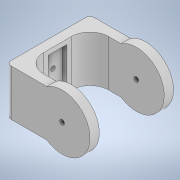
# Autodesk Inventor part: PartArm1
Saved by Autodesk Inventor 2022 (Build 260153000, 153)
## iProperties
Created: 2022-01-07
Part Number: PartArm1
Material: Generic
Document SubType Name: Modeling
Designer: nguye
Density: 1 g/cm^3
Appearance: Default
Author: nguye
Autodesk Inventor part; units mm, degrees
ref_plane "YZ Plane" through (0, 0, 0) normal (1, 0, 0) x (0, 1, 0)
ref_plane "XZ Plane" through (0, 0, 0) normal (0, 1, 0) x (-1, 0, 0)
ref_plane "XY Plane" through (0, 0, 0) normal (0, 0, 1) x (1, 0, 0)
sketch "Sketch1" plane through (0, 0, 0) normal (0, 1, 0) x (-1, 0, 0)
  line L0 (45, 0) -> (45, -45)
  line L1 (45, -45) -> (0, -45)
  line L2 (-45, 0) -> (-45, -45)
  line L3 (-45, -45) -> (0, -45)
  line L4 (45, 0) -> (45, 45)
  line L5 (45, 45) -> (0, 45)
  line L6 (-45, 0) -> (-45, 45)
  line L7 (-45, 45) -> (0, 45)
  line L8 (-45, 45) -> (-45, 35)
  line L9 (-45, 35) -> (51.6203, 35)
  line L10 (-45, -45) -> (-45, -35)
  line L11 (-45, -35) -> (58.872, -35)
  line L12 (45, 45) -> (35, 45)
  line L13 (35, 45) -> (35, -45)
  point P0 (0, 0)
  point P1 (35, 35)
  point P2 (35, -35)
  dimension "d0" = 45
  dimension "d1" = 45
  dimension "d2" = 10
  dimension "d3" = 10
  dimension "d4" = 10
  constraints: 28 end point, 4 point on line, 3 perpendicular
  measures "d0" distance of L0.end L1.end
  measures "d1" distance of L0.start L0.end
  measures "d2" distance of L7.start L8.end
  measures "d3" distance of L2.end L10.end
  measures "d4" distance of L4.end L12.end
extrude "Extrusion1" add sketch "Sketch1" along normal blind 60 contours L0 L11 L13 L9 L4 | L0 L1 L13 L11 | L9 L13 L5 L4 | L13 L1 L3 L2 L11 | L9 L6 L7 L5 L13
fillet "Fillet1" radius 20 2 edges at (-35, 30, 35) (-35, 30, -35)
fillet "Fillet2" radius 5 2 edges at (-45, 30, 45) (-45, 30, -45)
sketch "Sketch2" plane through (45, 0, -45) normal (0, 0, -1) x (-1, 0, 0)
  line L0 (0, 0) -> (0, 60) projected
  arc A0 (46.5831, 55) -> (46.5831, 5) centre (30, 30) ccw
  line L1 (90, 5) -> (46.5831, 5)
  line L2 (46.5831, 55) -> (90, 55)
  line L3 (90, 60) -> (90, 0) projected
  line L4 (60, 0) -> (0, 0) projected
  line L5 (90, 60) -> (0, 60)
  line L6 (0, 60) -> (0, 0)
  line L7 (0, 0) -> (90, 0)
  line L8 (90, 0) -> (90, 60)
  point P0 (45, 0)
  point P1 (30, 60)
  point P2 (30, 0)
  point P3 (0, 30)
  dimension "d10" = 5
  constraints: 12 end point, 3 parallel, 2 horizontal, 2 point on circle, 1 centre point, 1 perpendicular
  measures "d10" distance of L3.end L1.start
extrude "Extrusion2" cut sketch "Sketch2" against normal blind 161.25 contours L0 A0 L4 | L0 L5 A0 | A0 L1 L3 L7 L4 | L5 L3 L2 A0
sketch "Sketch3" plane through (-1.5831, 5, -45) normal (0, 0, -1) x (-1, 0, 0)
  line L0 (13.4169, 50) -> (0, 50) projected
  arc A0 (0, 50) -> (0, 0) centre (-16.5831, 25) ccw projected
  circle A1 centre (-16.5831, 25) radius 2.5
  point P0 (-1.5831, -5)
  dimension "d15" = 5
  constraints: 1 centre point, 1 coincident
  measures "d15" diameter of A1
extrude "Extrusion3" cut sketch "Sketch3" against normal blind 161.25
sketch "Sketch4" plane through (-45, 5, 40) normal (-1, 0, 0) x (0, 0, 1)
  circle A0 centre (-40, 25) radius 2.5
  point P0 (-40, -5)
  dimension "d18" = 5
  constraints: 1 centre point
  measures "d18" diameter of A0
extrude "Extrusion4" cut sketch "Sketch4" against normal blind 161.25
sketch "Sketch5" plane through (-45, 5, 40) normal (-1, 0, 0) x (0, 0, 1)
  point P0 (-40, -5)
sketch "Sketch6" plane through (-35, 5, -15) normal (1, 0, 0) x (0, 0, -1)
  line L0 (-15, 45) -> (-5, 45)
  line L1 (-5, 45) -> (-5, 5)
  line L2 (-5, 5) -> (-25, 5)
  line L3 (-25, 5) -> (-25, 45)
  line L4 (-25, 45) -> (-15, 45)
  point P0 (-15, -5)
  point P1 (-15, 25)
  dimension "d21" = 20
  dimension "d22" = 10
  dimension "d23" = 40
  dimension "d24" = 20
  dimension "d25" = 40
  dimension "d26" = 90
  constraints: 10 end point, 3 perpendicular
  measures "d21" distance of point (-15, 25) L0.start
  measures "d22" distance of L0.start L0.end
  measures "d23" distance of L0.end L1.end
  measures "d24" distance of L1.end L2.end
  measures "d25" distance of L2.end L3.end
  measures "d26" angle of L2 L3
extrude "Extrusion5" cut sketch "Sketch6" against normal blind 5
body "Solid1"
